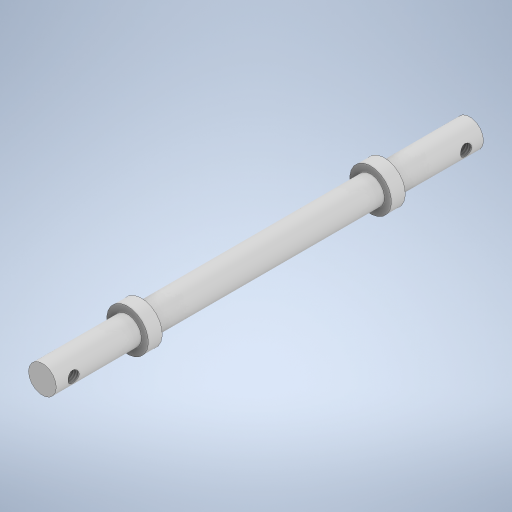
# Autodesk Inventor part: as1
Saved by Autodesk Inventor 2023 (Build 270158000, 158)
## iProperties
Created: 2022-12-05
Part Number: as1
Material: Generic
Document SubType Name: Modeling
Designer: daarn
Density: 1 g/cm^3
Appearance: Default
Author: daarn
Autodesk Inventor part; units mm, degrees
ref_plane "YZ Plane" through (0, 0, 0) normal (1, 0, 0) x (0, 1, 0)
ref_plane "XY Plane" through (0, 0, 0) normal (0, 0, 1) x (1, 0, 0)
sketch "Sketch1" plane through (0, 0, 0) normal (0, 0, 1) x (1, 0, 0)
  circle A0 centre (0, 0) radius 4
  dimension "d0" = 8
  constraints: 1 centre point, 1 coincident
  measures "d0" diameter of A0
extrude "Extrusion1" add sketch "Sketch1" along normal blind 123.051
sketch "Sketch3" plane through (0, 0, 0) normal (1, 0, 0) x (0, 1, 0)
  line L0 (4, 123.051) -> (-4, 123.051) projected
  point P0 (0, 0)
  point P1 (0, 5)
  point P2 (0, 118.051)
  dimension "d14" = 5
  dimension "d15" = 5
  dimension "d16" = 113.051
  constraints: 1 vertical alignment
  measures "d14" distance of point (0, 5) point (0, 0)
  measures "d15" distance from line of L0 point (0, 118.051)
  measures "d16" distance of point (0, 5) point (0, 118.051)
hole "Hole2" at (0, 0, 5) at (0, 0, 118.051) direction (1, 0, 0) diameter 3.242 depth 11.8 thread size "M4x0.7" class "6H" standard "ISO Metric profile"
sketch "Sketch4" plane through (0, 0, 0) normal (1, 0, 0) x (0, 1, 0)
  line L0 (4, 0) -> (4, 123.051) projected
  line L1 (4, 98.5255) -> (6, 98.5255)
  line L2 (6, 98.5255) -> (6, 94.5255)
  line L3 (6, 94.5255) -> (4, 94.5255)
  line L4 (4, 28.5255) -> (6, 28.5255)
  line L5 (6, 28.5255) -> (6, 24.5255)
  line L6 (6, 24.5255) -> (4, 24.5255)
  line L7 (4, 98.5255) -> (4, 94.5255)
  line L8 (4, 28.5255) -> (4, 24.5255)
  line L9 (0, -24.6102) -> (0, 147.6612) projected
  point P0 (0, 0)
  point P1 (5, 28.5255)
  point P2 (5, 94.5255)
  dimension "d24" = 66
  dimension "d25" = 4
  dimension "d26" = 4
  dimension "d27" = 24.5255
  dimension "d28" = 2
  dimension "d29" = 2
  constraints: 16 end point, 6 perpendicular, 4 point on line, 2 collinear, 2 midpoint
  measures "d24" distance of point (5, 28.526) point (5, 94.526)
  measures "d25" distance between parallel lines of L3 L1
  measures "d26" distance between parallel lines of L6 L4
  measures "d27" distance from line of point (0, 0) L6
  measures "d28" distance between parallel lines of L0 L5
  measures "d29" distance between parallel lines of L0 L2
revolve "Revolution1" add sketch "Sketch4" angle 360 about axis through (0, 0, -10) along (0, 0, 1)
ref_plane "Work Plane1" through (0, 0, 0) normal (0.7071, 0.7071, 0) x (0, 0, 1)
sketch "Sketch5" plane through (0, 0, 0) normal (0.7071, 0.7071, 0) x (0, 0, 1)
  circle A0 centre (26.5255, 0) radius 2
  circle A1 centre (96.5255, 0) radius 2
  line L0 (98.5255, -4) -> (98.5255, 4) projected
  line L1 (24.5255, 4) -> (24.5255, -4) projected
  point P0 (0, 0)
  dimension "d32" = 4
  dimension "d33" = 4
  constraints: 2 centre point, 2 horizontal alignment, 2 tangent
  measures "d32" diameter of A0
  measures "d33" diameter of A1
extrude "Extrusion2" cut sketch "Sketch5" against normal blind 10
body "Solid1"
